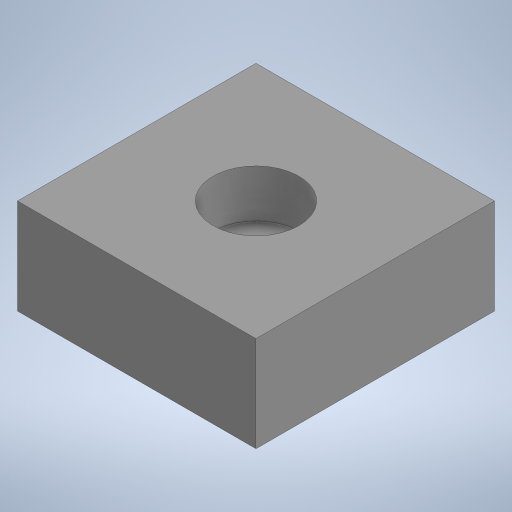
# Autodesk Inventor part: Base of Landing Docks
Saved by Autodesk Inventor 2023 (Build 270158000, 158)
## iProperties
Created: 2023-02-15
Part Number: Base of Landing Docks
Material: PLA 33 Plastic
Document SubType Name: Modeling
Designer: mihal
Density: 0.4135 g/cm^3
Appearance: Generic
Author: mihal
Autodesk Inventor part; units mm, degrees
ref_plane "YZ Plane" through (0, 0, 0) normal (1, 0, 0) x (0, 1, 0)
ref_plane "XZ Plane" through (0, 0, 0) normal (0, 1, 0) x (-1, 0, 0)
ref_plane "XY Plane" through (0, 0, 0) normal (0, 0, 1) x (1, 0, 0)
sketch "Sketch1" plane through (0, 0, 0) normal (0, 1, 0) x (-1, 0, 0)
  line L0 (0, 0) -> (50, 0)
  line L1 (50, 0) -> (50, -50)
  line L2 (50, -50) -> (0, -50)
  line L3 (0, -50) -> (0, 0)
  dimension "d0" = 50
  dimension "d1" = 50
  constraints: 8 end point, 2 parallel, 1 horizontal, 1 perpendicular
  measures "d0" distance of L1.end L2.end
  measures "d1" distance of L0.end L1.end
extrude "Extrusion1" add sketch "Sketch1" along normal blind 20
sketch "Sketch2" plane through (0, 20, 0) normal (0, 1, 0) x (1, 0, 0)
  line L0 (0, 50) -> (-50, 50) projected
  line L1 (-50, 50) -> (-50, 0) projected
  line L2 (-50, 0) -> (0, 0) projected
  line L3 (0, 0) -> (0, 50) projected
  line L4 (-25, 0) -> (-25, 50) construction
  line L5 (-50, 25) -> (0, 25) construction
  circle A0 centre (-25, 25) radius 9
  line L6 (-7.5, 26.25) -> (-42.5, 26.25)
  line L7 (-42.5, 26.25) -> (-42.5, 23.75)
  line L8 (-42.5, 23.75) -> (-7.5, 23.75)
  line L9 (-7.5, 23.75) -> (-7.5, 26.25)
  line L10 (-7.5, 26.25) -> (-42.5, 23.75) construction
  line L11 (-42.5, 26.25) -> (-7.5, 23.75) construction
  point P0 (-33.9128, 23.75)
  point P1 (-33.9128, 26.25)
  point P2 (-16.0872, 26.25)
  point P3 (-16.0872, 23.75)
  dimension "d4" = 18
  dimension "d7" = 35
  dimension "d8" = 2.5
  constraints: 16 end point, 7 midpoint, 2 parallel, 1 centre point, 1 horizontal, 1 perpendicular
  measures "d4" diameter of A0
  measures "d7" distance of L8.end L7.end
  measures "d8" distance of L7.end L6.end
extrude "Extrusion2" cut sketch "Sketch2" against normal blind 10 contours A0 L8 L6 | L6 A0 | A0 L8
body "Solid1"
